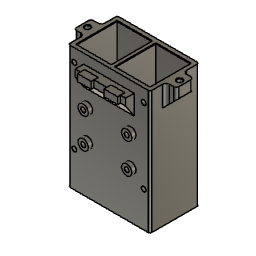
Battery v16 (Autodesk Fusion 360 design; units mm, degrees)
Autodesk Fusion 360 part; units mm, degrees
sketch "Battery" plane through (0, 0, 0) normal (0, 0, 1) x (1, 0, 0)
  line L0 (0, 0) -> (40, 0)
  line L1 (40, 0) -> (40, 47)
  line L2 (40, 47) -> (0, 47)
  line L3 (0, 47) -> (0, 0)
  line L4 (45, -0.2771) -> (85, -0.2771)
  line L5 (85, -0.2771) -> (85, 46.7229)
  line L6 (85, 46.7229) -> (45, 46.7229)
  line L7 (45, 46.7229) -> (45, -0.2771)
  dimension "d1" = 47
  dimension "d2" = 40
  dimension "d3" = 5
  constraint horizontal L0
  constraint vertical L1
  constraint horizontal L2
  constraint vertical L3
  constraint coincident L0.start L3.end
  constraint horizontal L4
  constraint vertical L5
  constraint horizontal L6
  constraint vertical L7
  constraint equal L3 L7
  constraint equal L0 L4
  measures "d1" distance of L0.start L2.end
  measures "d2" distance of L0.start L0.end
  measures "d3" horizontal distance of L0.end L4.start
extrude "Battery (1)" add sketch "Battery" along normal blind 138 makes body 1 at (0, 31.3333, 46) makes body 2 at (45, 31.0562, 46)
sketch "Base Box" plane through (0, 0, 0) normal (0, 0, -1) x (1, 0, 0)
  line L0 (0, 0) -> (0, -47)
  line L1 (0, -47) -> (40, -47)
  line L2 (40, -47) -> (40, 0)
  line L3 (40, 0) -> (0, 0)
  line L4 (-5, 5) -> (90, 5)
  line L5 (90, 5) -> (90, -52)
  line L6 (90, -52) -> (-5, -52)
  line L7 (-5, -52) -> (-5, 5)
  line L8 (85, 0.2771) -> (85, -46.7229)
  dimension "d6" = 5
  dimension "d7" = 5
  dimension "d8" = 5
  dimension "d9" = 5
  constraint horizontal L4
  constraint vertical L5
  constraint horizontal L6
  constraint vertical L7
  measures "d6" distance of L4.end L8
  measures "d7" horizontal distance of L0.start L4.start
  measures "d8" distance of L0.end L6
  measures "d9" distance of L0.start L4
extrude "Box Base" add sketch "Base Box" along normal blind 5 separate body contours L0 L1 L2 L3 | L4 L5 L6 L7 makes body 3
extrude "Extrude3" add 1 faces at (26.6667, 14, 0) along direction (0, 0, 1) up to surface (138 mm away) on bodies 3 bodies 3
combine "Combine1" operation cut target body 3 tool bodies 2 1 keep tools
ref_plane "WorkPlane1" through (42.5, 23.5, 66.5) normal (1, 0, 0) x (0, -1, 0)
sketch "Thumb Screw set" plane through (0, 0, 138) normal (0, 0, 1) x (-1, 0, 0)
  line L0 (0, -47) -> (-40, -47)
  line L1 (-40, -47) -> (-40, 0)
  line L2 (-40, 0) -> (0, 0)
  line L3 (0, 0) -> (0, -47)
  line L4 (-45, -46.7229) -> (-85, -46.7229)
  line L5 (-85, -46.7229) -> (-85, 0.2771)
  line L6 (-85, 0.2771) -> (-45, 0.2771)
  line L7 (-45, 0.2771) -> (-45, -46.7229)
  line L8 (-90, 5) -> (-90, -52)
  line L9 (-90, -52) -> (5, -52)
  line L10 (5, -52) -> (5, 5)
  line L11 (5, 5) -> (-90, 5)
  line L12 (-90, -13.5) -> (-102, -13.5)
  line L13 (-102, -13.5) -> (-102, -33.5)
  line L14 (-102, -33.5) -> (-90, -33.5)
  line L15 (-90, -33.5) -> (-90, -13.5)
  line L16 (-90, -33.5) -> (-90, -52) construction
  line L17 (-90, -13.5) -> (-90, 5) construction
  line L18 (-102, -23.5) -> (-90, -23.5) construction
  dimension "d20" = 12
  dimension "d30" = 20
  constraint horizontal L12
  constraint horizontal L14
  constraint vertical L15
  constraint coincident L8 L12.start
  constraint coincident L8.end L9.start
  constraint perpendicular L9 L16
  constraint coincident L8.start L11.end
  constraint perpendicular L11 L17
  constraint equal L16 L17
  constraint equal L12 L14
  constraint midpoint L13 L18.start
  constraint midpoint L15 L18.end
  measures "d20" distance of L12.start L12.end
  measures "d30" distance of L12.end L13.end
extrude "Thumb Screw set (1)" add sketch "Thumb Screw set" against normal blind 12 contours L8 L12 L13 L14 L15 bodies 3
chamfer "Chamfer1" distance 12 angle 45 1 edges at (90, 23.5, 126) on bodies 3
sketch "M4 screw/HS Clearance hole " plane through (0, 0, 138) normal (0, 0, 1) x (-1, 0, 0)
  line L0 (-90, -13.5) -> (-102, -13.5)
  line L1 (-102, -13.5) -> (-102, -33.5)
  line L2 (-102, -33.5) -> (-90, -33.5)
  circle A0 centre (-96, -23.5) radius 2
  circle A1 centre (-96, -23.5) radius 2.85
  line L3 (0, -47) -> (-40, -47)
  line L4 (-40, -47) -> (-40, 0)
  line L5 (-40, 0) -> (0, 0)
  line L6 (0, 0) -> (0, -47)
  line L7 (-45, -46.7229) -> (-85, -46.7229)
  line L8 (-85, -46.7229) -> (-85, 0.2771)
  line L9 (-85, 0.2771) -> (-45, 0.2771)
  line L10 (-45, 0.2771) -> (-45, -46.7229)
  line L11 (-90, -33.5) -> (-90, -52)
  line L12 (-90, -52) -> (5, -52)
  line L13 (5, -52) -> (5, 5)
  line L14 (5, 5) -> (-90, 5)
  line L15 (-90, 5) -> (-90, -13.5)
  line L16 (-102, -23.5) -> (-90, -23.5)
  dimension "d24" = 4
  dimension "d26" = 5.7
  constraint concentric A0 A1
  measures "d24" diameter of A0
  measures "d26" diameter of A1
extrude "Extrude5" cut sketch "M4 screw/HS Clearance hole " against normal through all contours A0 L16 | A0 L16 bodies 3
extrude "M4 HS Clearnace Hole" cut sketch "M4 screw/HS Clearance hole " against normal blind 8 contours A0 A1 L16 | A0 A1 L16 bodies 3
mirror "Mirror1" about plane through (42.5, 23.5, 66.5) normal (1, 0, 0) of bodies 3 merged
chamfer "Chamfer2" distance 0.6 angle 45 2 edges at (-13.6571, 22.4694, 138) (98.6571, 22.4694, 138) on bodies 3
chamfer "Chamfer3" distance 0.6 angle 45 8 edges at (0, 23.3615, 138) (20, 46.7229, 138) (40, 23.3615, 138) (20, 0, 138) (45, 23.3615, 138) (65, 46.7229, 138) (65, 0, 138) (85, 23.3615, 138) on bodies 3
fillet "Fillet1" radius 2 4 edges at (90, -5, 66.5) (90, 52, 66.5) (-5, -5, 66.5) (-5, 52, 66.5) on bodies 3
fillet "Fillet2" radius 3 4 edges at (102, 33.5, 132) (102, 13.5, 132) (-17, 33.5, 132) (-17, 13.5, 132) on bodies 3
fillet "Fillet3" radius 4 4 edges at (-5, 13.5, 126) (90, 13.5, 126) (90, 33.5, 126) (-5, 33.5, 126) on bodies 3
sketch "Tie Down" plane through (0, 0, 138) normal (0, 0, 1) x (-1, 0, 0)
  arc A0 (17, -16.5) -> (14, -13.5) centre (14, -16.5) ccw
  line L0 (14, -13.5) -> (9, -13.5)
  line L1 (-94, -13.5) -> (-99, -13.5)
  arc A1 (-99, -13.5) -> (-102, -16.5) centre (-99, -16.5) ccw
  line L2 (-102, -16.5) -> (-102, -30.5)
  arc A2 (-102, -30.5) -> (-99, -33.5) centre (-99, -30.5) ccw
  line L3 (-99, -33.5) -> (-94, -33.5)
  line L4 (9, -33.5) -> (14, -33.5)
  arc A3 (14, -33.5) -> (17, -30.5) centre (14, -30.5) ccw
  line L5 (17, -30.5) -> (17, -16.5)
  circle A4 centre (-96, -23.5) radius 3.45
  circle A5 centre (11, -23.5) radius 3.45
  line L6 (9, -33.5) -> (14, -33.5)
  line L7 (-99, -13.5) -> (-94, -13.5)
  arc A6 (17, -16.5) -> (14, -13.5) centre (14, -16.5) ccw
  circle A7 centre (11, -23.5) radius 2
  line L8 (17, -30.5) -> (17, -16.5)
  arc A8 (14, -33.5) -> (17, -30.5) centre (14, -30.5) ccw
  line L9 (14, -13.5) -> (9, -13.5)
  arc A9 (-99, -13.5) -> (-102, -16.5) centre (-99, -16.5) ccw
  arc A10 (-102, -30.5) -> (-99, -33.5) centre (-99, -30.5) ccw
  line L10 (-94, -33.5) -> (-99, -33.5)
  line L11 (-102, -30.5) -> (-102, -16.5)
  circle A11 centre (-96, -23.5) radius 2
  line L12 (9, -13.5) -> (-94, -13.5)
  line L13 (-94, -33.5) -> (9, -33.5)
  circle A12 centre (11, -23.5) radius 2.25
  circle A13 centre (-96, -23.5) radius 2.25
  dimension "d50" = 4.5
  constraint coincident L0.end L9.end
  constraint coincident L1.start L7.end
  constraint coincident L3.end L10.start
  constraint coincident L4.start L6.start
  constraint concentric A5 A12
  constraint concentric A11 A13
  constraint equal A12 A13
  measures "d50" diameter of A12
extrude "Extrude9" add sketch "Tie Down" along normal blind 5 separate body contours A0 L0 L1 A1 L2 A2 L3 L4 A3 L5 L6 L7 A6 L8 A8 L9 A9 A10 L10 L11 L12 L13 | A4 | A5 makes body 4
chamfer "Chamfer4" distance 0.6 angle 45 2 edges at (-8.9023, 22.6864, 143) (98.0977, 22.6864, 143) on bodies 4
fillet "Fillet4" radius 1 8 edges at (42.5, 13.5, 143) (101.1213, 14.3787, 143) (102, 23.5, 143) (101.1213, 32.6213, 143) (42.5, 33.5, 143) (-16.1213, 32.6213, 143) (-17, 23.5, 143) (-16.1213, 14.3787, 143) on bodies 4
ref_plane "WorkPlane2" through (42.5, -10, 66.5) normal (0, -1, 0) x (-1, 0, 0)
sketch "Sketch14" plane through (0, -10, 0) normal (0, -1, 0) x (-1, 0, 0)
  line L0 (-88, 5) -> (3, 5) construction
  line L1 (-88, -138) -> (3, -138) construction
  line L2 (-42.5, 5) -> (-42.5, -138) construction
  line L3 (-71, -89) -> (-14, -89)
  line L4 (-14, -89) -> (-14, -47)
  line L5 (-14, -47) -> (-71, -47)
  line L6 (-71, -47) -> (-71, -89)
  line L7 (-71, -89) -> (-14, -47) construction
  line L8 (-14, -89) -> (-71, -47) construction
  point P0 (-42.5, 5)
  point P1 (-42.5, -68)
  dimension "d63" = 42
  dimension "d64" = 57
  dimension "d65" = 70
  constraint midpoint L0 P0
  constraint coincident P0 L2.start
  constraint midpoint L1 L2.end
  constraint horizontal L3
  constraint perpendicular L3 L4
  constraint parallel L3 L5
  constraint parallel L4 L6
  constraint coincident L7 P1
  constraint coincident L8 P1
  constraint coincident L2 P1
  measures "d63" distance of L3.start L5.end
  measures "d64" distance of L4.end L5.end
  measures "d65" distance of L1 P1
sketch "Sketch15" plane through (42.5, -10, 68) normal (0, -1, 0) x (-1, 0, 0)
extrude "Extrude10" add sketch "Sketch14" along normal blind 30 separate body makes body 5
sketch "Sketch16" plane through (0, -40, 0) normal (0, -1, 0) x (1, 0, 0)
  line L0 (71, 47) -> (71, 89)
  line L1 (71, 89) -> (14, 89)
  line L2 (14, 89) -> (14, 47)
  line L3 (14, 47) -> (71, 47)
  line L4 (42.5, 47) -> (42.5, 89) construction
  line L5 (69.25, 87) -> (15.75, 87) construction
  line L6 (15.75, 87) -> (15.75, 49) construction
  line L7 (15.75, 49) -> (69.25, 49) construction
  line L8 (69.25, 49) -> (69.25, 87) construction
  line L9 (69.25, 87) -> (15.75, 49) construction
  line L10 (15.75, 87) -> (69.25, 49) construction
  circle A0 centre (17.25, 85.5) radius 1.5
  circle A1 centre (67.75, 85.5) radius 1.5
  circle A2 centre (17.25, 50.5) radius 1.5
  circle A3 centre (67.75, 50.5) radius 1.5
  point P0 (42.5, 68)
  dimension "d31" = 4
  dimension "d32" = 5.7
  dimension "d68" = 53.5
  dimension "d69" = 38
  dimension "d70" = 3
  constraint midpoint L3 L4.start
  constraint midpoint L1 L4.end
  constraint horizontal L5
  constraint perpendicular L5 L6
  constraint parallel L5 L7
  constraint parallel L6 L8
  constraint coincident L9 P0
  constraint coincident L10 P0
  constraint midpoint L4 P0
  constraint equal A0 A1
  constraint equal A0 A3
  constraint equal A0 A2
  constraint tangent L5 A0
  constraint tangent L6 A0
  constraint tangent L6 A2
  constraint tangent L7 A2
  constraint tangent L7 A3
  constraint tangent L8 A3
  constraint tangent L8 A1
  constraint tangent L5 A1
  measures "d68" distance of L6.end L7.end
  measures "d69" distance of L5.start L7.end
  measures "d70" diameter of A0
extrude "Extrude11" cut sketch "Sketch16" against normal up to surface (40 mm away) contours A0 | A1 | A2 | A3 bodies 3 5
sketch "Sketch17" plane through (0, -5, 0) normal (0, -1, 0) x (1, 0, 0)
  circle A0 centre (17.25, 85.5) radius 1.5
  circle A1 centre (17.25, 50.5) radius 1.5
  circle A2 centre (67.75, 85.5) radius 1.5
  circle A3 centre (67.75, 50.5) radius 1.5
  line L0 (-3, 138) -> (-3, -5)
  line L1 (-3, -5) -> (88, -5)
  line L2 (88, -5) -> (88, 138)
  line L3 (88, 138) -> (-3, 138)
  circle A4 centre (17.25, 85.5) radius 6
  circle A5 centre (67.75, 85.5) radius 6
  circle A6 centre (67.75, 50.5) radius 6
  circle A7 centre (17.25, 50.5) radius 6
  dimension "d73" = 12
  constraint concentric A0 A4
  constraint concentric A2 A5
  constraint concentric A3 A6
  constraint concentric A1 A7
  constraint equal A6 A7
  constraint equal A4 A7
  constraint equal A5 A7
  measures "d73" diameter of A7
extrude "Extrude12" add sketch "Sketch17" along normal up to surface (4.9 mm away) contours A4 | A5 | A6 | A7 bodies 3
sketch "Sketch18" plane through (0, -9.9, 0) normal (0, -1, 0) x (1, 0, 0)
  circle A0 centre (17.25, 85.5) radius 1.5 construction
  circle A1 centre (17.25, 85.5) radius 6 construction
  circle A2 centre (17.25, 85.5) radius 2.6
  circle A3 centre (17.25, 50.5) radius 1.5 construction
  circle A4 centre (67.75, 50.5) radius 1.5 construction
  circle A5 centre (67.75, 85.5) radius 1.5 construction
  circle A6 centre (17.25, 50.5) radius 2.6
  circle A7 centre (67.75, 50.5) radius 2.6
  circle A8 centre (67.75, 85.5) radius 2.6
  dimension "d76" = 5.2
  constraint concentric A0 A2
  constraint concentric A3 A6
  constraint concentric A4 A7
  constraint concentric A5 A8
  constraint equal A2 A8
  constraint equal A6 A7
  constraint equal A2 A6
  measures "d76" diameter of A2
extrude "Extrude13" cut sketch "Sketch18" against normal blind 3.8 bodies 3
chamfer "Chamfer5" distance 0.2 angle 45 4 edges at (65.3259, -9.9, 86.4402) (65.3259, -9.9, 51.4402) (14.8259, -9.9, 51.4402) (14.8259, -9.9, 86.4402) on bodies 3
ref_plane "WorkPlane3" through (42.5, -25, 119) normal (0, 0, 1) x (-1, 0, 0)
sketch "Sketch20" plane through (0, 0, 119) normal (0, 0, 1) x (1, 0, 0)
  line L0 (71, -10) -> (14, -10) construction
  line L1 (19, -10) -> (34.8, -10)
  line L2 (34.8, -10) -> (34.8, -18.2)
  line L3 (34.8, -18.2) -> (19, -18.2)
  line L4 (19, -18.2) -> (19, -10)
  line L5 (49.8, -10) -> (65.6, -10)
  line L6 (65.6, -10) -> (65.6, -18.2)
  line L7 (65.6, -18.2) -> (49.8, -18.2)
  line L8 (49.8, -18.2) -> (49.8, -10)
  line L9 (14, -10) -> (14, -40)
  dimension "d83" = 8.2
  dimension "d84" = 15.8
  dimension "d85" = 15
  dimension "d86" = 5
  constraint horizontal L1
  constraint vertical L2
  constraint horizontal L3
  constraint vertical L4
  constraint coincident L0 L1.start
  constraint horizontal L5
  constraint vertical L6
  constraint horizontal L7
  constraint vertical L8
  constraint coincident L0 L5.start
  constraint equal L3 L7
  constraint equal L2 L8
  measures "d83" distance of L1.start L3.end
  measures "d84" distance of L2.end L3.end
  measures "d85" distance of L2 L8
  measures "d86" distance of L4 L9
extrude "Extrude14" add sketch "Sketch20" along normal blind 8 separate body makes body 6 at (29.5333, -12.7333, 119) makes body 7 at (60.3333, -12.7333, 119)
sketch "Sketch21" plane through (0, -5, 0) normal (0, -1, 0) x (1, 0, 0)
  circle A0 centre (17.25, 50.5) radius 6
  circle A1 centre (17.25, 85.5) radius 6
  circle A2 centre (67.75, 50.5) radius 6
  circle A3 centre (67.75, 85.5) radius 6
  line L0 (-3, 138) -> (-3, -5)
  line L1 (-3, -5) -> (88, -5)
  line L2 (88, -5) -> (88, 138)
  line L3 (88, 138) -> (-3, 138)
  line L4 (19, 119) -> (34.8, 119) construction
  line L5 (34.8, 119) -> (34.8, 127) construction
  line L6 (34.8, 127) -> (19, 127) construction
  line L7 (19, 127) -> (19, 119) construction
  line L8 (49.8, 119) -> (65.6, 119) construction
  line L9 (65.6, 119) -> (65.6, 127) construction
  line L10 (65.6, 127) -> (49.8, 127) construction
  line L11 (49.8, 127) -> (49.8, 119) construction
  line L12 (13, 127) -> (71.6, 127)
  line L13 (71.6, 127) -> (71.6, 104)
  line L14 (71.6, 104) -> (13, 104)
  line L15 (13, 104) -> (13, 127)
  dimension "d89" = 6
  dimension "d90" = 6
  dimension "d91" = 15
  constraint horizontal L12
  constraint vertical L13
  constraint horizontal L14
  constraint vertical L15
  constraint coincident L6.end L12
  measures "d89" distance of L7 L15
  measures "d90" distance of L9 L13
  measures "d91" distance of L8.end L14
extrude "Extrude15" add sketch "Sketch21" along normal blind 10 separate body contours L12 L13 L14 L15 makes body 8
combine "Combine2" operation add target body 8 tool bodies 3
combine "Combine3" operation cut target body 8 tool bodies 7 6 keep tools
chamfer "Chamfer6" distance 15 distance2 10 1 edges at (42.3, -15, 104) measured on face at (39.8, -15, 109) on bodies 8
sketch "Sketch22" plane through (0, -5, 0) normal (0, -1, 0) x (1, 0, 0)
  line L0 (-3, 138) -> (-3, -5)
  line L1 (-3, -5) -> (88, -5)
  line L2 (88, -5) -> (88, 138)
  line L3 (88, 138) -> (-3, 138)
  circle A0 centre (67.75, 85.5) radius 6
  circle A1 centre (67.75, 50.5) radius 6
  circle A2 centre (17.25, 85.5) radius 6
  circle A3 centre (17.25, 50.5) radius 6
  line L4 (13, 104) -> (13, 127)
  line L5 (13, 127) -> (71.6, 127)
  line L6 (71.6, 127) -> (71.6, 104)
  line L7 (71.6, 104) -> (13, 104)
  line L8 (-2, 32) -> (86.6, 32)
  line L9 (86.6, 32) -> (86.6, 127)
  line L10 (86.6, 127) -> (-2, 127)
  line L11 (-2, 127) -> (-2, 32)
  line L12 (14, 47) -> (71, 47)
  line L13 (13, 104) -> (8, 104)
  line L14 (8, 104) -> (8, 39)
  line L15 (8, 39) -> (76.6, 39)
  line L16 (76.6, 39) -> (76.6, 104)
  line L17 (76.6, 104) -> (71.6, 104)
  line L18 (2, 123) -> (82.6, 123) construction
  line L19 (82.6, 123) -> (82.6, 36) construction
  line L20 (82.6, 36) -> (2, 36) construction
  line L21 (2, 36) -> (2, 123) construction
  circle A4 centre (2, 123) radius 1.5
  circle A5 centre (82.6, 123) radius 1.5
  circle A6 centre (82.6, 36) radius 1.5
  circle A7 centre (2, 36) radius 1.5
  dimension "d96" = 15
  dimension "d97" = 15
  dimension "d98" = 15
  dimension "d99" = 5
  dimension "d100" = 65
  dimension "d101" = 4
  dimension "d102" = 4
  dimension "d103" = 4
  dimension "d104" = 4
  dimension "d105" = 3
  constraint horizontal L8
  constraint vertical L9
  constraint horizontal L10
  constraint vertical L11
  constraint coincident L4.end L10
  constraint coincident L4.start L7.end
  constraint perpendicular L4 L13
  constraint perpendicular L8 L14
  constraint perpendicular L14 L15
  constraint perpendicular L15 L16
  constraint coincident L6.end L7.start
  constraint perpendicular L6 L17
  constraint equal L13 L17
  constraint horizontal L18
  constraint vertical L19
  constraint horizontal L20
  constraint vertical L21
  constraint coincident L18.start L21.end
  constraint coincident L18.end L19.start
  constraint coincident L19.end L20.start
  constraint coincident L20.end L21.start
  constraint equal A6 A7
  constraint equal A5 A7
  constraint equal A4 A7
  measures "d96" distance of L8 L12
  measures "d97" distance of L4 L11
  measures "d98" distance of L5.end L9.end
  measures "d99" distance of L16.end L6.end
  measures "d100" distance of L15.end L16.end
  measures "d101" distance of L8 L20
  measures "d102" distance of L11 L21
  measures "d103" distance of L9 L19
  measures "d104" distance of L10 L18
  measures "d105" diameter of A7
extrude "Extrude16" cut sketch "Sketch22" against normal up to surface (5 mm away) contours A4 | A5 | A6 | A7 bodies 8
sketch "Sketch24" plane through (0, -5, 0) normal (0, -1, 0) x (1, 0, 0)
  circle A0 centre (82.6, 123) radius 1.5
  circle A1 centre (2, 123) radius 1.5
  circle A2 centre (82.6, 36) radius 1.5
  circle A3 centre (2, 36) radius 1.5
  line L0 (-3, 138) -> (-3, -5)
  line L1 (-3, -5) -> (88, -5)
  line L2 (88, -5) -> (88, 138)
  line L3 (88, 138) -> (-3, 138)
  circle A4 centre (67.75, 85.5) radius 6
  circle A5 centre (67.75, 50.5) radius 6
  circle A6 centre (17.25, 85.5) radius 6
  circle A7 centre (17.25, 50.5) radius 6
  line L4 (13, 104) -> (13, 127)
  line L5 (13, 127) -> (71.6, 127)
  line L6 (71.6, 127) -> (71.6, 104)
  line L7 (71.6, 104) -> (13, 104)
  circle A8 centre (2, 36) radius 2.6
  circle A9 centre (82.6, 36) radius 2.6
  circle A10 centre (82.6, 123) radius 2.6
  circle A11 centre (2, 123) radius 2.6
  dimension "d108" = 5.2
  constraint concentric A3 A8
  constraint concentric A2 A9
  constraint concentric A0 A10
  constraint concentric A1 A11
  constraint equal A10 A11
  constraint equal A8 A11
  constraint equal A9 A11
  measures "d108" diameter of A11
extrude "Extrude17" cut sketch "Sketch24" against normal blind 3.8 contours A8 | A9 | A10 | A11 bodies 8
chamfer "Chamfer7" distance 0.2 angle 45 4 edges at (-0.4241, -5, 36.9402) (80.1759, -5, 36.9402) (80.1759, -5, 123.9402) (-0.4241, -5, 123.9402) on bodies 8
extrude "Extrude18" add sketch "Sketch22" along normal blind 37.5 separate body contours L4 L6 L8 L9 L10 L11 L13 L14 L15 L16 L17 makes body 9
sketch "Sketch25" plane through (13, 0, 0) normal (1, 0, 0) x (0, 1, 0)
  line L0 (-5, 104) -> (-5, 127)
  line L1 (-5, 127) -> (-42.5, 127)
  line L2 (-42.5, 127) -> (-42.5, 104)
  line L3 (-42.5, 104) -> (-5, 104)
  line L4 (-15, 119) -> (-42.5, 119)
  line L5 (-42.5, 119) -> (-42.5, 127)
  line L6 (-42.5, 127) -> (-15, 127)
  line L7 (-15, 127) -> (-15, 119)
  point P0 (-15, 119)
  constraint horizontal L4
  constraint vertical L5
  constraint horizontal L6
  constraint vertical L7
  constraint coincident L1.end L2.start
  constraint coincident P0 L4.start
extrude "Extrude19" add sketch "Sketch25" along normal up to surface (58.6 mm away) separate body contours L1 L2 L4 L5 L6 L7 makes body 10
combine "Combine4" operation cut target body 10 tool bodies 6 7 keep tools
combine "Combine5" operation add target body 9 tool bodies 10
sketch "Sketch26" plane through (0, -42.5, 0) normal (0, -1, 0) x (1, 0, 0)
  line L0 (71.6, 119) -> (71.6, 104)
  line L1 (71.6, 104) -> (76.6, 104)
  line L2 (76.6, 104) -> (76.6, 39)
  line L3 (76.6, 39) -> (8, 39)
  line L4 (8, 39) -> (8, 104)
  line L5 (8, 104) -> (13, 104)
  line L6 (13, 104) -> (13, 119)
  line L7 (13, 119) -> (71.6, 119)
  circle A0 centre (2, 123) radius 1.5
  circle A1 centre (2, 36) radius 1.5
  circle A2 centre (82.6, 36) radius 1.5
  circle A3 centre (82.6, 123) radius 1.5
  line L8 (86.6, 127) -> (-2, 127)
  line L9 (-2, 127) -> (-2, 32)
  line L10 (-2, 32) -> (86.6, 32)
  line L11 (86.6, 32) -> (86.6, 127)
  line L12 (-2, 32) -> (86.6, 32)
  line L13 (86.6, 32) -> (86.6, 127)
  line L14 (86.6, 127) -> (-2, 127)
  line L15 (-2, 127) -> (-2, 32)
  constraint horizontal L12
  constraint vertical L13
  constraint horizontal L14
  constraint vertical L15
  constraint coincident L8.start L11.end
  constraint coincident L9.end L10.start
extrude "Extrude20" add sketch "Sketch26" along normal blind 5 contours L0 L1 L2 L3 L4 L5 L6 L7 | L8 L9 L10 L11 L12 L13 L14 L15 bodies 9
hidden bodies 1 2 4 5 9
equation "d3 = BoxOffset"
equation "d6 = BoxOffset"
equation "d7 = BoxOffset"
equation "d8 = BoxOffset"
equation "d9 = BoxOffset"
equation "BoxOffset = 5 mm"
equation "M4_HSL_W = 5.7 mm" comment "Width of M4 HS"
equation "M4_HSL_L = 8 mm"
equation "d26 = M4_HSL_W"
equation "d27 = -M4_HSL_L"
equation "d32 = M4_HSL_W"
equation "d76 = M3_S_D"
equation "M3_S_D = 5.2 mm"
equation "M3_S_L = 3.8 mm"
equation "d79 = -M3_S_L"
equation "d108 = M3_S_D"
equation "d109 = -M3_S_L"
named bodies: "Battery 1", "Battery 2", "Box Base", "Tie Down", "BMS", "xt 60 Left", "XT 60 right", "Box", "Cover"
